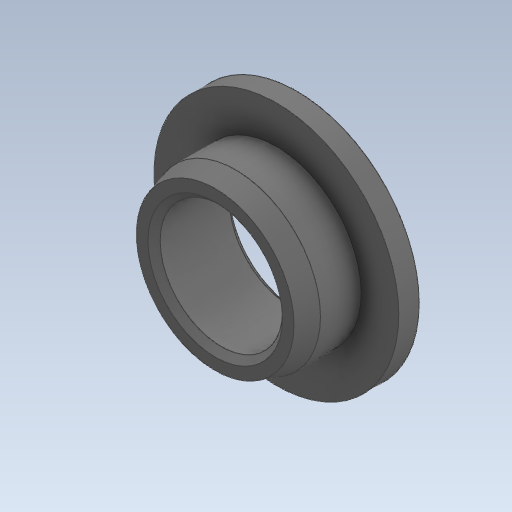
# Autodesk Inventor part: 80F-0603
Saved by Autodesk Inventor 2020.4 (Build 244396000, 396)
## iProperties
Part Number: 80F-0603
Material: 一般
Document SubType Name: Modeling
Designer: Masato Kubotera
Density: 1.18394 g/cm^3
Appearance: 灰色
Catalog Web Link: https://jp.misumi-ec.com/vona2/detail/221000090789/?HissuCode=80F-0603
Mass: 0.186667 g
Surface Area: 3.47407 cm^2
Volume: 0.157665 cm^3
Description: ReadyMade
Author: Masato Kubotera
Autodesk Inventor part; units mm, degrees
ref_plane "YZ Plane" through (0, 0, 0) normal (1, 0, 0) x (0, 1, 0)
ref_plane "XZ Plane" through (0, 0, 0) normal (0, 1, 0) x (-1, 0, 0)
ref_plane "XY Plane" through (0, 0, 0) normal (0, 0, 1) x (1, 0, 0)
sketch "スケッチ1" plane through (0, 0, 0) normal (0, 1, 0) x (-1, 0, 0)
  line L0 (-3, 0.3) -> (-3, 3.7)
  line L1 (-3.3, 4) -> (-3.8618, 4)
  line L2 (-4.1618, 3) -> (-4.1618, 1)
  line L3 (-4.1618, 1) -> (-6, 1)
  line L4 (-6, 1) -> (-6, 0)
  line L5 (-6, 0) -> (-3.3, 0)
  line L6 (-3, 3.7) -> (-3.3, 4)
  line L7 (-3, 0.3) -> (-3.3, 0)
  line L8 (-3.8618, 4) -> (-4.1618, 3)
  line L9 (0, -0.8) -> (0, 4.8) projected
  point P0 (0, 0)
  point P1 (-3, 0)
  point P2 (-3, 4)
  point P3 (-4.1618, 4)
  dimension "d0" = 4
  dimension "d1" = 6
  dimension "d2" = 1
  dimension "d3" = 0.3
  dimension "d4" = 0.3
  dimension "d5" = 0.3
  dimension "d6" = 0.3
  dimension "d7" = 3
  dimension "d8" = 0.3
  dimension "d9" = 1
  constraints: 18 end point, 6 point on line, 4 perpendicular, 1 parallel, 1 vertical
  measures "d0" distance of point (-3, 0) point (-3, 4)
  measures "d1" distance of point (0, 0) L4.end
  measures "d2" distance of L3.end L4.end
  measures "d3" distance of L0.end point (-3, 4)
  measures "d4" distance of L1.start point (-3, 4)
  measures "d5" distance of L0.start point (-3, 0)
  measures "d6" distance of L5.end point (-3, 0)
  measures "d7" distance of point (0, 0) point (-3, 0)
  measures "d8" distance of L1.end point (-4.162, 4)
  measures "d9" distance of L2.start point (-4.162, 4)
revolve "回転1" add sketch "スケッチ1" angle 360 about axis through (0, 0, -10) along (0, 0, 1)
equation "\"d4\" = d3"
equation "\"d5\" = d3"
equation "\"d6\" = d5"
equation "\"d8\" = d3"
